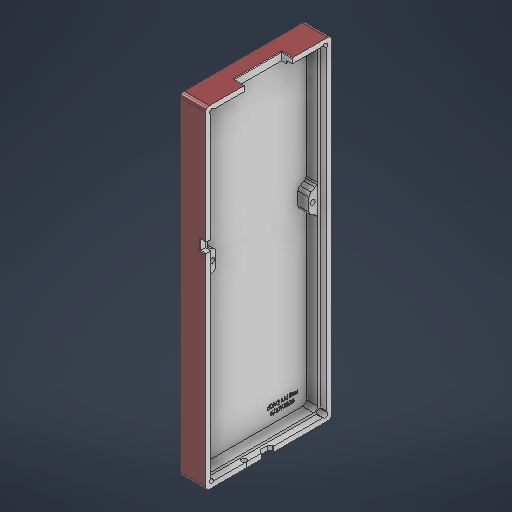
# Autodesk Inventor part: cDAQ_Box_Lid_v0.2
Saved by Autodesk Inventor 2027 (Build 310192000, 192)
## iProperties
Created: 2026-05-08
Part Number: cDAQ_Box_Lid_v0.2
Material: Generic
Document SubType Name: Modeling
Designer: giese
Density: 1 g/cm^3
Appearance: Default
Author: giese
Autodesk Inventor part; units mm, degrees
(part 1 of 2)
ref_plane "YZ Plane" through (0, 0, 0) normal (1, 0, 0) x (0, 1, 0)
ref_plane "XZ Plane" through (0, 0, 0) normal (0, 1, 0) x (-1, 0, 0)
ref_plane "XY Plane" through (0, 0, 0) normal (0, 0, 1) x (1, 0, 0)
sketch "Sketch1" plane through (0, 0, 0) normal (1, 0, 0) x (0, 1, 0)
  line L0 (50.7569, 48.4212) -> (-216.9591, 48.4212)
  line L1 (-216.9591, 48.4212) -> (-216.9591, -53.1788)
  line L2 (-216.9591, -53.1788) -> (50.7569, -53.1788)
  line L3 (50.7569, -53.1788) -> (50.7569, 48.4212)
  point P0 (0, 0)
  dimension "d0" = 101.6
  dimension "d1" = 267.716
  constraints: 8 end point, 2 parallel, 1 horizontal, 1 perpendicular
  measures "d0" distance of L2.end L0.start
  measures "d1" distance of L0.start L0.end
extrude "Extrusion1" add sketch "Sketch1" along normal blind 20.32
sketch "Sketch2" plane through (20.32, 0, 0) normal (1, 0, 0) x (0, 0, -1)
  line L0 (-42.0712, 44.4069) -> (46.8288, 44.4069)
  line L1 (46.8288, 44.4069) -> (46.8288, -210.6091)
  line L2 (46.8288, -210.6091) -> (-42.0712, -210.6091)
  line L3 (-42.0712, -210.6091) -> (-42.0712, 44.4069)
  line L4 (-48.4212, 50.7569) -> (-48.4212, -216.9591) projected
  line L5 (-48.4212, -216.9591) -> (53.1788, -216.9591) projected
  point P0 (0, 0)
  dimension "d4" = 88.9
  dimension "d5" = 255.016
  dimension "d6" = 6.35
  dimension "d7" = 6.35
  constraints: 8 end point, 2 parallel, 1 horizontal, 1 perpendicular
  measures "d4" distance of L0.start L0.end
  measures "d5" distance of L0.end L1.end
  measures "d6" distance between parallel lines of L4 L3
  measures "d7" distance between parallel lines of L5 L2
extrude "Extrusion2" cut sketch "Sketch2" against normal blind 13.97
sketch "Sketch3" plane through (0, 0, 0) normal (-1, 0, 0) x (0, 0, 1)
  circle A0 centre (-30.3188, 7.3229) radius 2
  line L0 (-53.1788, -216.9591) -> (-53.1788, 50.7569) projected
  line L1 (-53.1788, 50.7569) -> (48.4212, 50.7569) projected
  circle A1 centre (-11.82, 7.3229) radius 2
  circle A2 centre (6.6789, 7.3229) radius 2
  point P0 (0, 0)
  dimension "d10" = 22.86
  dimension "d11" = 43.434
  dimension "d12" = 43.434
  dimension "d13" = 18.4988
  dimension "d14" = 4
  dimension "d15" = 4
  dimension "d16" = 43.434
  dimension "d17" = 18.4988
  dimension "d18" = 36.9976
  dimension "d21" = 4
  constraints: 3 centre point
  measures "d10" distance from line of L0 A0.centre
  measures "d11" distance from line of L1 A0.centre
  measures "d12" distance from line of L1 A1.centre
  measures "d13" distance of A0.centre A1.centre
  measures "d14" diameter of A1
  measures "d15" diameter of A2
  measures "d16" distance from line of L1 A2.centre
  measures "d17" distance of A1.centre A2.centre
  measures "d18" distance of A0.centre A2.centre
  measures "d21" diameter of A0
extrude "Extrusion3" [suppressed]
sketch "Sketch6" plane through (0, 50.7569, 48.4212) normal (0, 1, 0) x (1, 0, 0)
  line L0 (20.32, 6.35) -> (20.32, 95.25) projected
  line L1 (11.684, 31.75) -> (20.32, 31.75)
  line L2 (20.32, 31.75) -> (20.32, 69.85)
  line L3 (20.32, 69.85) -> (11.684, 69.85)
  line L4 (11.684, 69.85) -> (11.684, 31.75)
  line L5 (0, 101.6) -> (20.32, 101.6) projected
  point P0 (0, 48.4212)
  point P1 (16.002, 69.85)
  point P2 (16.002, 31.75)
  dimension "d30" = 8.636
  dimension "d31" = 38.1
  dimension "d32" = 31.75
  constraints: 8 end point, 2 midpoint, 2 parallel, 1 horizontal, 1 perpendicular, 1 point on line
  measures "d30" distance between parallel lines of L0 L4
  measures "d31" distance of point (16.002, 69.85) point (16.002, 31.75)
  measures "d32" distance between parallel lines of L5 L3
extrude "Extrusion5" cut sketch "Sketch6" against normal blind 6.35
fillet "Fillet1" radius 3.175 4 edges at (10.16, 50.7569, -53.1788) (10.16, 50.7569, 48.4212) (10.16, -216.9591, 48.4212) (10.16, -216.9591, -53.1788)
sketch "Sketch7" plane through (20.32, 0, 0) normal (1, 0, 0) x (0, 0, -1)
  line L0 (-42.0712, -210.6091) -> (-42.0712, 44.4069) projected
  line L1 (-42.0712, 44.4069) -> (-42.3252, 44.4069)
  line L2 (-42.3252, 46.5659) -> (-44.2302, 46.5659)
  line L3 (-44.2302, 46.5659) -> (-44.2302, 51.0109)
  line L4 (-42.0712, -190.1621) -> (-42.0712, -210.6091)
  line L5 (46.8288, -210.6091) -> (-42.0712, -210.6091) projected
  line L6 (-40.4202, -212.7681) -> (-44.2302, -212.7681)
  line L7 (-44.2302, -212.7681) -> (-44.2302, -190.1621)
  line L8 (46.8288, 44.4069) -> (46.8288, -210.6091) projected
  line L9 (46.8288, -192.7021) -> (46.8288, -210.6091)
  line L10 (46.8288, -210.6091) -> (43.9078, -210.6091)
  line L11 (46.8288, -210.6091) -> (46.8288, -192.7021)
  line L12 (48.9878, -192.7021) -> (48.9878, -212.7681)
  line L13 (48.9878, -212.7681) -> (43.9078, -212.7681)
  line L14 (-42.0712, 44.4069) -> (46.8288, 44.4069) projected
  line L15 (42.0028, 44.4069) -> (46.8288, 44.4069)
  line L16 (48.9878, 48.4709) -> (48.9878, 46.5659)
  line L17 (48.9878, 46.5659) -> (42.0028, 46.5659)
  line L18 (-42.3252, 46.5659) -> (42.0028, 46.5659)
  line L19 (42.0028, 44.4069) -> (-42.3252, 44.4069)
  line L20 (48.9878, 48.4709) -> (48.9878, -192.7021)
  line L21 (44.2888, -195.2421) -> (44.2888, 44.4069)
  line L22 (43.9078, -210.6091) -> (-40.4202, -210.6091)
  line L23 (-40.4202, -212.7681) -> (43.9078, -212.7681)
  line L24 (-44.2302, -190.1621) -> (-44.2302, 51.0109)
  line L25 (-42.0712, 44.4069) -> (-42.0712, -190.1621)
  point P0 (0, 0)
  point P1 (-42.0712, 51.0109)
  point P2 (-44.2302, 48.9789)
  point P3 (46.8288, 48.4709)
  point P4 (48.9878, 46.5659)
  point P5 (-44.2302, 46.5659)
  dimension "d34" = 2.159
  dimension "d35" = 2.159
  dimension "d38" = 2.159
  dimension "d39" = 2.159
  dimension "d42" = 2.159
  dimension "d43" = 2.159
  dimension "d46" = 2.159
  dimension "d47" = 2.159
  constraints: 44 end point, 9 point on line, 4 parallel, 4 perpendicular, 2 collinear, 2 horizontal, 2 vertical
  measures "d34" distance between parallel lines of L2 L1
  measures "d35" distance between parallel lines of L0 L3
  measures "d38" distance between parallel lines of L7 L0
  measures "d39" distance between parallel lines of L5 L6
  measures "d42" distance between parallel lines of L5 L13
  measures "d43" distance between parallel lines of L8 L12
  measures "d46" distance between parallel lines of L14 L17
  measures "d47" distance between parallel lines of L8 L16
extrude "Extrusion6" cut sketch "Sketch7" against normal blind 5 contours L0 L14 L8 L5 | L18 L17 L20 L12 L13 L23 L6 L7 L24 L2
fillet "Fillet2" radius 3.175 6 edges at (10.835, 44.4069, 42.0712) (10.835, 44.4069, -46.8288) (10.835, -210.6091, 42.0712) (17.82, -212.7681, 44.2302) (10.835, -210.6091, -46.8288) (17.82, -212.7681, -48.9878)
sketch "Sketch11" plane through (15.32, 0, 0) normal (1, 0, 0) x (0, 0, -1)
  circle A0 centre (48.0988, 45.6769) radius 1.9939
  line L0 (50.0038, 50.7569) -> (21.4288, 50.7569) projected
  line L1 (53.1788, -213.7841) -> (53.1788, 47.5819) projected
  arc A1 (46.9238, 45.7719) -> (43.7488, 48.9469) centre (43.7488, 45.7719) ccw projected
  circle A2 centre (-43.3412, 45.6769) radius 1.9939
  line L2 (-48.4212, 47.5819) -> (-48.4212, -213.7841) projected
  line L3 (-16.6712, 50.7569) -> (-45.2462, 50.7569) projected
  circle A3 centre (48.0988, -211.8791) radius 1.9939
  line L4 (-45.2462, -216.9591) -> (50.0038, -216.9591) projected
  circle A4 centre (-43.3412, -211.8791) radius 1.9939
  circle A5 centre (43.0188, -63.5431) radius 1.9939
  circle A6 centre (-38.2612, -63.5431) radius 1.9939
  point P0 (0, 0)
  point P1 (45.9939, 48.017)
  point P2 (48.5528, -43.2993)
  point P3 (45.3778, -46.4743)
  point P4 (-30.4007, -42.8803)
  point P5 (-33.5757, -46.0553)
  dimension "d58" = 3.9878
  dimension "d59" = 5.08
  dimension "d60" = 5.08
  dimension "d61" = 3.9878
  dimension "d62" = 3.9878
  dimension "d63" = 5.08
  dimension "d64" = 5.08
  dimension "d65" = 3.9878
  dimension "d66" = 5.08
  dimension "d67" = 5.08
  dimension "d76" = 5.08
  dimension "d77" = 5.08
  dimension "d114" = 3.9878
  dimension "d115" = 114.3
  dimension "d116" = 10.16
  dimension "d117" = 3.9878
  dimension "d118" = 114.3
  dimension "d119" = 10.16
  constraints: 6 centre point, 1 point on circle
  measures "d58" diameter of A0
  measures "d59" distance from line of L2 A2.centre
  measures "d60" distance from line of L3 A2.centre
  measures "d61" diameter of A2
  measures "d62" diameter of A3
  measures "d63" distance from line of L1 A3.centre
  measures "d64" distance from line of L4 A3.centre
  measures "d65" diameter of A4
  measures "d66" distance from line of L2 A4.centre
  measures "d67" distance from line of L4 A4.centre
  measures "d76" distance from line of L1 A0.centre
  measures "d77" distance from line of L0 A0.centre
  measures "d114" diameter of A5
  measures "d115" distance from line of A5.centre L0
  measures "d116" distance from line of L1 A5.centre
  measures "d117" diameter of A6
  measures "d118" distance from line of A6.centre L3
  measures "d119" distance from line of L2 A6.centre
extrude "Extrusion8" cut sketch "Sketch11" along normal blind 5.08 and the other way blind 17.78
sketch "Sketch13" plane through (6.35, 0, 0) normal (1, 0, 0) x (0, 0, -1)
  line L0 (14.9448, -196.2811) -> (40.0007, -196.2811) construction
  line L1 (40.0007, -196.2811) -> (40.0007, -205.1454) construction
  line L2 (40.0007, -205.1454) -> (14.9448, -205.1454) construction
  line L3 (14.9448, -205.1454) -> (14.9448, -196.2811) construction
  spline S0 degree 2 poles (16.1329, -199.5168) (15.8958, -199.5168) (15.5031, -199.3711) (15.3623, -199.2229) knots 0 0 0 1 2 2 2
  spline S1 degree 2 poles (15.3623, -199.2229) (15.2215, -199.0772) (15.0659, -198.6276) (15.0659, -198.3263) knots 0 0 0 1 2 2 2
  spline S2 degree 2 poles (15.0659, -198.3263) (15.0659, -198.0249) (15.2264, -197.5853) (15.3623, -197.4371) knots 0 0 0 1 2 2 2
  spline S3 degree 2 poles (15.3623, -197.4371) (15.4981, -197.2864) (15.9007, -197.1258) (16.1329, -197.1258) knots 0 0 0 1 2 2 2
  spline S4 degree 2 poles (16.1329, -197.1258) (16.3206, -197.1258) (16.6714, -197.232) (16.8072, -197.3012) knots 0 0 0 1 2 2 2
  line L4 (16.8072, -197.3012) -> (16.8072, -197.7335)
  line L5 (16.8072, -197.7335) -> (16.785, -197.7335)
  spline S5 degree 2 poles (16.785, -197.7335) (16.743, -197.6989) (16.6146, -197.61) (16.5232, -197.563) knots 0 0 0 1 2 2 2
  spline S6 degree 2 poles (16.5232, -197.563) (16.4417, -197.5235) (16.2243, -197.4618) (16.1255, -197.4618) knots 0 0 0 1 2 2 2
  spline S7 degree 2 poles (16.1255, -197.4618) (15.8266, -197.4618) (15.4635, -197.9138) (15.4635, -198.3263) knots 0 0 0 1 2 2 2
  spline S8 degree 2 poles (15.4635, -198.3263) (15.4635, -198.7289) (15.8143, -199.1809) (16.1255, -199.1809) knots 0 0 0 1 2 2 2
  spline S9 degree 2 poles (16.1255, -199.1809) (16.3132, -199.1809) (16.6541, -199.0253) (16.785, -198.9043) knots 0 0 0 1 2 2 2
  line L6 (16.785, -198.9043) -> (16.8072, -198.9043)
  line L7 (16.8072, -198.9043) -> (16.8072, -199.3365)
  spline S10 degree 2 poles (16.8072, -199.3365) (16.7504, -199.3637) (16.5775, -199.4402) (16.5084, -199.4575) knots 0 0 0 1 2 2 2
  spline S11 degree 2 poles (16.5084, -199.4575) (16.4096, -199.4872) (16.2539, -199.5168) (16.1329, -199.5168) knots 0 0 0 1 2 2 2
  spline S12 degree 2 poles (19.5909, -197.9434) (19.5909, -198.3608) (19.2525, -199.0327) (18.9685, -199.2204) knots 0 0 0 1 2 2 2
  spline S13 degree 2 poles (18.9685, -199.2204) (18.7363, -199.3661) (18.2596, -199.4649) (17.8891, -199.4649) knots 0 0 0 1 2 2 2
  line L8 (17.8891, -199.4649) -> (17.1876, -199.4649)
  line L9 (17.1876, -199.4649) -> (17.1876, -196.4169)
  line L10 (17.1876, -196.4169) -> (17.8817, -196.4169)
  spline S14 degree 2 poles (17.8817, -196.4169) (18.3115, -196.4169) (18.8005, -196.5454) (18.9734, -196.659) knots 0 0 0 1 2 2 2
  spline S15 degree 2 poles (18.9734, -196.659) (19.2674, -196.8541) (19.5909, -197.4988) (19.5909, -197.9434) knots 0 0 0 1 2 2 2
  spline S16 degree 2 poles (19.1686, -197.9385) (19.1686, -197.5877) (18.9364, -197.0913) (18.7067, -196.9505) knots 0 0 0 1 2 2 2
  spline S17 degree 2 poles (18.7067, -196.9505) (18.5437, -196.8541) (18.1756, -196.7677) (17.9014, -196.7677) knots 0 0 0 1 2 2 2
  line L11 (17.9014, -196.7677) -> (17.5927, -196.7677)
  line L12 (17.5927, -196.7677) -> (17.5927, -199.1142)
  line L13 (17.5927, -199.1142) -> (17.9014, -199.1142)
  spline S18 degree 2 poles (17.9014, -199.1142) (18.1707, -199.1142) (18.5782, -199.0278) (18.7437, -198.9117) knots 0 0 0 1 2 2 2
  spline S19 degree 2 poles (18.7437, -198.9117) (18.9561, -198.7684) (19.1686, -198.2942) (19.1686, -197.9385) knots 0 0 0 1 2 2 2
  line L14 (19.7021, -199.4649) -> (20.7296, -196.4169)
  line L15 (20.7296, -196.4169) -> (21.2286, -196.4169)
  line L16 (21.2286, -196.4169) -> (22.2561, -199.4649)
  line L17 (22.2561, -199.4649) -> (21.8288, -199.4649)
  line L18 (21.8288, -199.4649) -> (21.5521, -198.6128)
  line L19 (21.5521, -198.6128) -> (20.3888, -198.6128)
  line L20 (20.3888, -198.6128) -> (20.1121, -199.4649)
  line L21 (20.1121, -199.4649) -> (19.7021, -199.4649)
  line L22 (21.441, -198.267) -> (20.9692, -196.8319)
  line L23 (20.9692, -196.8319) -> (20.4999, -198.267)
  line L24 (20.4999, -198.267) -> (21.441, -198.267)
  spline S20 degree 2 poles (25.0768, -200.2109) (24.9657, -200.2381) (24.7236, -200.2677) (24.6026, -200.2677) knots 0 0 0 1 2 2 2
  spline S21 degree 2 poles (24.6026, -200.2677) (24.2593, -200.2677) (23.832, -199.8848) (23.8122, -199.5292) knots 0 0 0 1 2 2 2
  spline S22 degree 2 poles (23.8122, -199.5292) (23.785, -199.5292) (23.7381, -199.5292) (23.7183, -199.5292) knots 0 0 0 1 2 2 2
  spline S23 degree 2 poles (23.7183, -199.5292) (23.4096, -199.5292) (22.9131, -199.3192) (22.7353, -199.1142) knots 0 0 0 1 2 2 2
  spline S24 degree 2 poles (22.7353, -199.1142) (22.5599, -198.9117) (22.3722, -198.3189) (22.3722, -197.9434) knots 0 0 0 1 2 2 2
  spline S25 degree 2 poles (22.3722, -197.9434) (22.3722, -197.5581) (22.5624, -196.9752) (22.7377, -196.7677) knots 0 0 0 1 2 2 2
  spline S26 degree 2 poles (22.7377, -196.7677) (22.9156, -196.5627) (23.4121, -196.3527) (23.7183, -196.3527) knots 0 0 0 1 2 2 2
  spline S27 degree 2 poles (23.7183, -196.3527) (24.0296, -196.3527) (24.5285, -196.5701) (24.7014, -196.7677) knots 0 0 0 1 2 2 2
  spline S28 degree 2 poles (24.7014, -196.7677) (24.8743, -196.9678) (25.067, -197.563) (25.067, -197.9434) knots 0 0 0 1 2 2 2
  spline S29 degree 2 poles (25.067, -197.9434) (25.067, -198.5362) (24.6051, -199.3069) (24.2025, -199.4427) knots 0 0 0 1 2 2 2
  spline S30 degree 2 poles (24.2025, -199.4427) (24.2123, -199.5563) (24.2716, -199.7391) (24.3185, -199.791) knots 0 0 0 1 2 2 2
  spline S31 degree 2 poles (24.3185, -199.791) (24.3754, -199.8552) (24.531, -199.9145) (24.6693, -199.9145) knots 0 0 0 1 2 2 2
  spline S32 degree 2 poles (24.6693, -199.9145) (24.7508, -199.9145) (24.9731, -199.8626) (25.0225, -199.8429) knots 0 0 0 1 2 2 2
  line L25 (25.0225, -199.8429) -> (25.0768, -199.8429)
  line L26 (25.0768, -199.8429) -> (25.0768, -200.2109)
  spline S33 degree 2 poles (24.6446, -197.9434) (24.6446, -197.6396) (24.5137, -197.1728) (24.3951, -197.0196) knots 0 0 0 1 2 2 2
  spline S34 degree 2 poles (24.3951, -197.0196) (24.2741, -196.8615) (23.9332, -196.7035) (23.7208, -196.7035) knots 0 0 0 1 2 2 2
  spline S35 degree 2 poles (23.7208, -196.7035) (23.501, -196.7035) (23.17, -196.8566) (23.044, -197.0196) knots 0 0 0 1 2 2 2
  spline S36 degree 2 poles (23.044, -197.0196) (22.923, -197.1752) (22.7945, -197.647) (22.7945, -197.9434) knots 0 0 0 1 2 2 2
  spline S37 degree 2 poles (22.7945, -197.9434) (22.7945, -198.5436) (23.2984, -199.1834) (23.7208, -199.1834) knots 0 0 0 1 2 2 2
  spline S38 degree 2 poles (23.7208, -199.1834) (24.1432, -199.1834) (24.6446, -198.5436) (24.6446, -197.9434) knots 0 0 0 1 2 2 2
  line L27 (28.5867, -199.4649) -> (26.8207, -199.4649)
  line L28 (26.8207, -199.4649) -> (26.8207, -196.4169)
  line L29 (26.8207, -196.4169) -> (27.2258, -196.4169)
  line L30 (27.2258, -196.4169) -> (27.2258, -199.1043)
  line L31 (27.2258, -199.1043) -> (28.5867, -199.1043)
  line L32 (28.5867, -199.1043) -> (28.5867, -199.4649)
  line L33 (29.2685, -199.4649) -> (28.8831, -199.4649)
  line L34 (28.8831, -199.4649) -> (28.8831, -197.1777)
  line L35 (28.8831, -197.1777) -> (29.2685, -197.1777)
  line L36 (29.2685, -197.1777) -> (29.2685, -199.4649)
  line L37 (29.2956, -196.7973) -> (28.8584, -196.7973)
  line L38 (28.8584, -196.7973) -> (28.8584, -196.3972)
  line L39 (28.8584, -196.3972) -> (29.2956, -196.3972)
  line L40 (29.2956, -196.3972) -> (29.2956, -196.7973)
  line L41 (31.5927, -199.4649) -> (31.2074, -199.4649)
  line L42 (31.2074, -199.4649) -> (31.2074, -199.2328)
  spline S39 degree 2 poles (31.2074, -199.2328) (31.1185, -199.3069) (30.9876, -199.4057) (30.8987, -199.4477) knots 0 0 0 1 2 2 2
  spline S40 degree 2 poles (30.8987, -199.4477) (30.8172, -199.4872) (30.6418, -199.5292) (30.5257, -199.5292) knots 0 0 0 1 2 2 2
  spline S41 degree 2 poles (30.5257, -199.5292) (30.338, -199.5292) (30.0218, -199.3736) (29.9107, -199.2229) knots 0 0 0 1 2 2 2
  spline S42 degree 2 poles (29.9107, -199.2229) (29.7995, -199.0722) (29.676, -198.6276) (29.676, -198.3386) knots 0 0 0 1 2 2 2
  spline S43 degree 2 poles (29.676, -198.3386) (29.676, -198.0373) (29.8316, -197.5976) (29.9675, -197.4321) knots 0 0 0 1 2 2 2
  spline S44 degree 2 poles (29.9675, -197.4321) (30.0934, -197.2839) (30.4467, -197.1135) (30.6418, -197.1135) knots 0 0 0 1 2 2 2
  spline S45 degree 2 poles (30.6418, -197.1135) (30.8122, -197.1135) (31.0666, -197.1901) (31.2074, -197.2691) knots 0 0 0 1 2 2 2
  line L43 (31.2074, -197.2691) -> (31.2074, -196.2811)
  line L44 (31.2074, -196.2811) -> (31.5927, -196.2811)
  line L45 (31.5927, -196.2811) -> (31.5927, -199.4649)
  line L46 (31.2074, -198.9092) -> (31.2074, -197.5877)
  spline S46 degree 2 poles (31.2074, -197.5877) (31.0642, -197.5186) (30.8369, -197.4667) (30.706, -197.4667) knots 0 0 0 1 2 2 2
  spline S47 degree 2 poles (30.706, -197.4667) (30.4096, -197.4667) (30.0737, -197.9113) (30.0737, -198.3312) knots 0 0 0 1 2 2 2
  spline S48 degree 2 poles (30.0737, -198.3312) (30.0737, -198.7363) (30.3306, -199.1636) (30.6146, -199.1636) knots 0 0 0 1 2 2 2
  spline S49 degree 2 poles (30.6146, -199.1636) (30.7653, -199.1636) (31.0716, -199.0253) (31.2074, -198.9092) knots 0 0 0 1 2 2 2
  spline S50 degree 2 poles (35.5571, -198.5288) (35.5571, -198.756) (35.3842, -199.1043) (35.241, -199.2179) knots 0 0 0 1 2 2 2
  spline S51 degree 2 poles (35.241, -199.2179) (35.0681, -199.3513) (34.6753, -199.4649) (34.3641, -199.4649) knots 0 0 0 1 2 2 2
  line L47 (34.3641, -199.4649) -> (33.4897, -199.4649)
  line L48 (33.4897, -199.4649) -> (33.4897, -196.4169)
  line L49 (33.4897, -196.4169) -> (34.2974, -196.4169)
  spline S52 degree 2 poles (34.2974, -196.4169) (34.6235, -196.4169) (34.9495, -196.4589) (35.0977, -196.5404) knots 0 0 0 1 2 2 2
  spline S53 degree 2 poles (35.0977, -196.5404) (35.2632, -196.6269) (35.4139, -196.9109) (35.4139, -197.1036) knots 0 0 0 1 2 2 2
  spline S54 degree 2 poles (35.4139, -197.1036) (35.4139, -197.3185) (35.1866, -197.6594) (34.9865, -197.7557) knots 0 0 0 1 2 2 2
  line L50 (34.9865, -197.7557) -> (34.9865, -197.7705)
  spline S55 degree 2 poles (34.9865, -197.7705) (35.2583, -197.8446) (35.5571, -198.2373) (35.5571, -198.5288) knots 0 0 0 1 2 2 2
  spline S56 degree 2 poles (35.1347, -198.5461) (35.1347, -198.3732) (35.0359, -198.1509) (34.8877, -198.0719) knots 0 0 0 1 2 2 2
  spline S57 degree 2 poles (34.8877, -198.0719) (34.7914, -198.0225) (34.5642, -197.9928) (34.3542, -197.9928) knots 0 0 0 1 2 2 2
  line L51 (34.3542, -197.9928) -> (33.8948, -197.9928)
  line L52 (33.8948, -197.9928) -> (33.8948, -199.1191)
  line L53 (33.8948, -199.1191) -> (34.2233, -199.1191)
  spline S58 degree 2 poles (34.2233, -199.1191) (34.4901, -199.1191) (34.7964, -199.0697) (34.9149, -198.9907) knots 0 0 0 1 2 2 2
  spline S59 degree 2 poles (34.9149, -198.9907) (35.0285, -198.9092) (35.1347, -198.7066) (35.1347, -198.5461) knots 0 0 0 1 2 2 2
  spline S60 degree 2 poles (34.9915, -197.1604) (34.9915, -197.0517) (34.9174, -196.8887) (34.8359, -196.8418) knots 0 0 0 1 2 2 2
  spline S61 degree 2 poles (34.8359, -196.8418) (34.7371, -196.7874) (34.4975, -196.7627) (34.2826, -196.7627) knots 0 0 0 1 2 2 2
  line L54 (34.2826, -196.7627) -> (33.8948, -196.7627)
  line L55 (33.8948, -196.7627) -> (33.8948, -197.6544)
  line L56 (33.8948, -197.6544) -> (34.3542, -197.6544)
  spline S62 degree 2 poles (34.3542, -197.6544) (34.5444, -197.6544) (34.7247, -197.6149) (34.8211, -197.5532) knots 0 0 0 1 2 2 2
  spline S63 degree 2 poles (34.8211, -197.5532) (34.9149, -197.4939) (34.9915, -197.3037) (34.9915, -197.1604) knots 0 0 0 1 2 2 2
  spline S64 degree 2 poles (37.8098, -198.3213) (37.8098, -198.8993) (37.254, -199.5292) (36.7897, -199.5292) knots 0 0 0 1 2 2 2
  spline S65 degree 2 poles (36.7897, -199.5292) (36.3129, -199.5292) (35.7671, -198.8796) (35.7671, -198.3213) knots 0 0 0 1 2 2 2
  spline S66 degree 2 poles (35.7671, -198.3213) (35.7671, -197.7483) (36.3302, -197.1135) (36.7897, -197.1135) knots 0 0 0 1 2 2 2
  spline S67 degree 2 poles (36.7897, -197.1135) (37.254, -197.1135) (37.8098, -197.7458) (37.8098, -198.3213) knots 0 0 0 1 2 2 2
  spline S68 degree 2 poles (37.4121, -198.3213) (37.4121, -197.8767) (37.0885, -197.4445) (36.7897, -197.4445) knots 0 0 0 1 2 2 2
  spline S69 degree 2 poles (36.7897, -197.4445) (36.4908, -197.4445) (36.1647, -197.8767) (36.1647, -198.3213) knots 0 0 0 1 2 2 2
  spline S70 degree 2 poles (36.1647, -198.3213) (36.1647, -198.7536) (36.4908, -199.1982) (36.7897, -199.1982) knots 0 0 0 1 2 2 2
  spline S71 degree 2 poles (36.7897, -199.1982) (37.0861, -199.1982) (37.4121, -198.761) (37.4121, -198.3213) knots 0 0 0 1 2 2 2
  line L57 (39.9809, -199.4649) -> (39.5091, -199.4649)
  line L58 (39.5091, -199.4649) -> (38.9534, -198.6054)
  line L59 (38.9534, -198.6054) -> (38.3828, -199.4649)
  line L60 (38.3828, -199.4649) -> (37.9456, -199.4649)
  line L61 (37.9456, -199.4649) -> (38.7385, -198.3312)
  line L62 (38.7385, -198.3312) -> (37.953, -197.1777)
  line L63 (37.953, -197.1777) -> (38.4248, -197.1777)
  line L64 (38.4248, -197.1777) -> (38.9781, -198.0299)
  line L65 (38.9781, -198.0299) -> (39.5437, -197.1777)
  line L66 (39.5437, -197.1777) -> (39.9809, -197.1777)
  line L67 (39.9809, -197.1777) -> (39.193, -198.3065)
  line L68 (39.193, -198.3065) -> (39.9809, -199.4649)
  spline S72 degree 2 poles (20.0133, -203.4954) (20.0133, -203.73) (19.8577, -204.1277) (19.7268, -204.2611) knots 0 0 0 1 2 2 2
  spline S73 degree 2 poles (19.7268, -204.2611) (19.5909, -204.4019) (19.2501, -204.5476) (19.0451, -204.5476) knots 0 0 0 1 2 2 2
  spline S74 degree 2 poles (19.0451, -204.5476) (18.8401, -204.5476) (18.5017, -204.4093) (18.3732, -204.271) knots 0 0 0 1 2 2 2
  spline S75 degree 2 poles (18.3732, -204.271) (18.2151, -204.1055) (18.0373, -203.5497) (18.0373, -203.1446) knots 0 0 0 1 2 2 2
  spline S76 degree 2 poles (18.0373, -203.1446) (18.0373, -202.747) (18.2003, -202.1072) (18.3707, -201.8701) knots 0 0 0 1 2 2 2
  spline S77 degree 2 poles (18.3707, -201.8701) (18.5362, -201.6379) (19.0599, -201.3786) (19.4032, -201.3786) knots 0 0 0 1 2 2 2
  spline S78 degree 2 poles (19.4032, -201.3786) (19.5045, -201.3786) (19.6823, -201.3983) (19.749, -201.4206) knots 0 0 0 1 2 2 2
  line L69 (19.749, -201.4206) -> (19.749, -201.8133)
  line L70 (19.749, -201.8133) -> (19.7317, -201.8133)
  spline S79 degree 2 poles (19.7317, -201.8133) (19.6749, -201.7837) (19.4674, -201.7318) (19.3489, -201.7318) knots 0 0 0 1 2 2 2
  spline S80 degree 2 poles (19.3489, -201.7318) (18.9685, -201.7318) (18.5017, -202.2456) (18.4572, -202.7494) knots 0 0 0 1 2 2 2
  spline S81 degree 2 poles (18.4572, -202.7494) (18.6029, -202.6482) (18.9092, -202.537) (19.092, -202.537) knots 0 0 0 1 2 2 2
  spline S82 degree 2 poles (19.092, -202.537) (19.2698, -202.537) (19.5366, -202.6087) (19.6823, -202.7173) knots 0 0 0 1 2 2 2
  spline S83 degree 2 poles (19.6823, -202.7173) (19.8503, -202.8433) (20.0133, -203.2336) (20.0133, -203.4954) knots 0 0 0 1 2 2 2
  spline S84 degree 2 poles (19.5983, -203.5127) (19.5983, -203.325) (19.4995, -203.0705) (19.3909, -202.9816) knots 0 0 0 1 2 2 2
  spline S85 degree 2 poles (19.3909, -202.9816) (19.3094, -202.9174) (19.1068, -202.8754) (19.0006, -202.8754) knots 0 0 0 1 2 2 2
  spline S86 degree 2 poles (19.0006, -202.8754) (18.8573, -202.8754) (18.5881, -202.9619) (18.4572, -203.0434) knots 0 0 0 1 2 2 2
  spline S87 degree 2 poles (18.4572, -203.0434) (18.4547, -203.0878) (18.4498, -203.1718) (18.4498, -203.236) knots 0 0 0 1 2 2 2
  spline S88 degree 2 poles (18.4498, -203.236) (18.4498, -203.5522) (18.5733, -203.94) (18.6672, -204.0413) knots 0 0 0 1 2 2 2
  spline S89 degree 2 poles (18.6672, -204.0413) (18.7536, -204.1376) (18.9413, -204.2142) (19.0475, -204.2142) knots 0 0 0 1 2 2 2
  spline S90 degree 2 poles (19.0475, -204.2142) (19.2945, -204.2142) (19.5983, -203.8634) (19.5983, -203.5127) knots 0 0 0 1 2 2 2
  line L71 (21.6411, -201.2995) -> (20.448, -205.1454)
  line L72 (20.448, -205.1454) -> (20.1022, -205.1454)
  line L73 (20.1022, -205.1454) -> (21.2903, -201.2995)
  line L74 (21.2903, -201.2995) -> (21.6411, -201.2995)
  line L75 (23.7035, -204.4834) -> (22.2166, -204.4834)
  line L76 (22.2166, -204.4834) -> (22.2166, -204.1722)
  line L77 (22.2166, -204.1722) -> (22.7698, -204.1722)
  line L78 (22.7698, -204.1722) -> (22.7698, -202.1295)
  line L79 (22.7698, -202.1295) -> (22.2166, -202.1295)
  line L80 (22.2166, -202.1295) -> (22.2166, -201.8504)
  spline S91 degree 2 poles (22.2166, -201.8504) (22.5303, -201.8504) (22.8267, -201.6725) (22.8464, -201.4255) knots 0 0 0 1 2 2 2
  line L81 (22.8464, -201.4255) -> (23.1626, -201.4255)
  line L82 (23.1626, -201.4255) -> (23.1626, -204.1722)
  line L83 (23.1626, -204.1722) -> (23.7035, -204.1722)
  line L84 (23.7035, -204.1722) -> (23.7035, -204.4834)
  line L85 (26.1785, -201.8923) -> (24.8595, -204.4834)
  line L86 (24.8595, -204.4834) -> (24.4248, -204.4834)
  line L87 (24.4248, -204.4834) -> (25.8178, -201.7935)
  line L88 (25.8178, -201.7935) -> (24.2444, -201.7935)
  line L89 (24.2444, -201.7935) -> (24.2444, -201.4354)
  line L90 (24.2444, -201.4354) -> (26.1785, -201.4354)
  line L91 (26.1785, -201.4354) -> (26.1785, -201.8923)
  line L92 (27.8186, -201.2995) -> (26.6255, -205.1454)
  line L93 (26.6255, -205.1454) -> (26.2797, -205.1454)
  line L94 (26.2797, -205.1454) -> (27.4678, -201.2995)
  line L95 (27.4678, -201.2995) -> (27.8186, -201.2995)
  line L96 (30.0342, -204.4834) -> (28.1545, -204.4834)
  line L97 (28.1545, -204.4834) -> (28.1545, -204.0511)
  spline S92 degree 2 poles (28.1545, -204.0511) (28.357, -203.861) (28.7176, -203.5077) (28.8905, -203.3175) knots 0 0 0 1 2 2 2
  spline S93 degree 2 poles (28.8905, -203.3175) (29.2388, -202.9347) (29.4932, -202.4753) (29.4932, -202.2307) knots 0 0 0 1 2 2 2
  spline S94 degree 2 poles (29.4932, -202.2307) (29.4932, -202.1023) (29.4142, -201.9096) (29.3426, -201.8479) knots 0 0 0 1 2 2 2
  spline S95 degree 2 poles (29.3426, -201.8479) (29.2709, -201.7861) (29.0832, -201.7244) (28.9696, -201.7244) knots 0 0 0 1 2 2 2
  spline S96 degree 2 poles (28.9696, -201.7244) (28.8609, -201.7244) (28.6386, -201.7787) (28.5373, -201.8207) knots 0 0 0 1 2 2 2
  spline S97 degree 2 poles (28.5373, -201.8207) (28.4509, -201.8553) (28.2903, -201.9541) (28.2409, -201.9887) knots 0 0 0 1 2 2 2
  line L98 (28.2409, -201.9887) -> (28.2187, -201.9887)
  line L99 (28.2187, -201.9887) -> (28.2187, -201.554)
  spline S98 degree 2 poles (28.2187, -201.554) (28.3447, -201.4922) (28.7967, -201.3712) (28.9992, -201.3712) knots 0 0 0 1 2 2 2
  spline S99 degree 2 poles (28.9992, -201.3712) (29.4265, -201.3712) (29.9082, -201.8232) (29.9082, -202.2085) knots 0 0 0 1 2 2 2
  spline S100 degree 2 poles (29.9082, -202.2085) (29.9082, -202.3888) (29.8242, -202.6902) (29.7501, -202.8186) knots 0 0 0 1 2 2 2
  spline S101 degree 2 poles (29.7501, -202.8186) (29.676, -202.952) (29.4611, -203.2138) (29.3426, -203.3398) knots 0 0 0 1 2 2 2
  spline S102 degree 2 poles (29.3426, -203.3398) (29.1499, -203.5497) (28.6781, -203.9993) (28.5373, -204.1302) knots 0 0 0 1 2 2 2
  line L100 (28.5373, -204.1302) -> (30.0342, -204.1302)
  line L101 (30.0342, -204.1302) -> (30.0342, -204.4834)
  spline S103 degree 2 poles (32.3387, -202.9594) (32.3387, -203.7794) (31.862, -204.5476) (31.3655, -204.5476) knots 0 0 0 1 2 2 2
  spline S104 degree 2 poles (31.3655, -204.5476) (30.8616, -204.5476) (30.3898, -203.7646) (30.3898, -202.9619) knots 0 0 0 1 2 2 2
  spline S105 degree 2 poles (30.3898, -202.9619) (30.3898, -202.1369) (30.8666, -201.3736) (31.3655, -201.3736) knots 0 0 0 1 2 2 2
  spline S106 degree 2 poles (31.3655, -201.3736) (31.8669, -201.3736) (32.3387, -202.1641) (32.3387, -202.9594) knots 0 0 0 1 2 2 2
  spline S107 degree 2 poles (31.815, -203.8881) (31.8743, -203.7375) (31.9237, -203.2731) (31.9237, -202.9594) knots 0 0 0 1 2 2 2
  spline S108 degree 2 poles (31.9237, -202.9594) (31.9237, -202.6457) (31.8743, -202.1838) (31.8126, -202.0282) knots 0 0 0 1 2 2 2
  spline S109 degree 2 poles (31.8126, -202.0282) (31.7508, -201.8726) (31.5359, -201.712) (31.3655, -201.712) knots 0 0 0 1 2 2 2
  spline S110 degree 2 poles (31.3655, -201.712) (31.1951, -201.712) (30.9752, -201.8726) (30.911, -202.0331) knots 0 0 0 1 2 2 2
  spline S111 degree 2 poles (30.911, -202.0331) (30.8493, -202.1888) (30.8048, -202.663) (30.8048, -202.9619) knots 0 0 0 1 2 2 2
  spline S112 degree 2 poles (30.8048, -202.9619) (30.8048, -203.283) (30.8443, -203.7128) (30.9086, -203.8807) knots 0 0 0 1 2 2 2
  spline S113 degree 2 poles (30.9086, -203.8807) (30.9678, -204.0388) (31.1877, -204.2092) (31.3655, -204.2092) knots 0 0 0 1 2 2 2
  spline S114 degree 2 poles (31.3655, -204.2092) (31.5335, -204.2092) (31.7533, -204.0487) (31.815, -203.8881) knots 0 0 0 1 2 2 2
  line L102 (34.6086, -204.4834) -> (32.729, -204.4834)
  line L103 (32.729, -204.4834) -> (32.729, -204.0511)
  spline S115 degree 2 poles (32.729, -204.0511) (32.9315, -203.861) (33.2921, -203.5077) (33.465, -203.3175) knots 0 0 0 1 2 2 2
  spline S116 degree 2 poles (33.465, -203.3175) (33.8133, -202.9347) (34.0677, -202.4753) (34.0677, -202.2307) knots 0 0 0 1 2 2 2
  spline S117 degree 2 poles (34.0677, -202.2307) (34.0677, -202.1023) (33.9887, -201.9096) (33.917, -201.8479) knots 0 0 0 1 2 2 2
  spline S118 degree 2 poles (33.917, -201.8479) (33.8454, -201.7861) (33.6577, -201.7244) (33.5441, -201.7244) knots 0 0 0 1 2 2 2
  spline S119 degree 2 poles (33.5441, -201.7244) (33.4354, -201.7244) (33.2131, -201.7787) (33.1118, -201.8207) knots 0 0 0 1 2 2 2
  spline S120 degree 2 poles (33.1118, -201.8207) (33.0254, -201.8553) (32.8648, -201.9541) (32.8154, -201.9887) knots 0 0 0 1 2 2 2
  line L104 (32.8154, -201.9887) -> (32.7932, -201.9887)
  line L105 (32.7932, -201.9887) -> (32.7932, -201.554)
  spline S121 degree 2 poles (32.7932, -201.554) (32.9191, -201.4922) (33.3712, -201.3712) (33.5737, -201.3712) knots 0 0 0 1 2 2 2
  spline S122 degree 2 poles (33.5737, -201.3712) (34.001, -201.3712) (34.4827, -201.8232) (34.4827, -202.2085) knots 0 0 0 1 2 2 2
  spline S123 degree 2 poles (34.4827, -202.2085) (34.4827, -202.3888) (34.3987, -202.6902) (34.3246, -202.8186) knots 0 0 0 1 2 2 2
  spline S124 degree 2 poles (34.3246, -202.8186) (34.2505, -202.952) (34.0356, -203.2138) (33.917, -203.3398) knots 0 0 0 1 2 2 2
  spline S125 degree 2 poles (33.917, -203.3398) (33.7244, -203.5497) (33.2526, -203.9993) (33.1118, -204.1302) knots 0 0 0 1 2 2 2
  line L106 (33.1118, -204.1302) -> (34.6086, -204.1302)
  line L107 (34.6086, -204.1302) -> (34.6086, -204.4834)
  spline S126 degree 2 poles (36.9428, -203.4954) (36.9428, -203.73) (36.7872, -204.1277) (36.6563, -204.2611) knots 0 0 0 1 2 2 2
  spline S127 degree 2 poles (36.6563, -204.2611) (36.5204, -204.4019) (36.1796, -204.5476) (35.9746, -204.5476) knots 0 0 0 1 2 2 2
  spline S128 degree 2 poles (35.9746, -204.5476) (35.7695, -204.5476) (35.4312, -204.4093) (35.3027, -204.271) knots 0 0 0 1 2 2 2
  spline S129 degree 2 poles (35.3027, -204.271) (35.1446, -204.1055) (34.9668, -203.5497) (34.9668, -203.1446) knots 0 0 0 1 2 2 2
  spline S130 degree 2 poles (34.9668, -203.1446) (34.9668, -202.747) (35.1298, -202.1072) (35.3002, -201.8701) knots 0 0 0 1 2 2 2
  spline S131 degree 2 poles (35.3002, -201.8701) (35.4657, -201.6379) (35.9894, -201.3786) (36.3327, -201.3786) knots 0 0 0 1 2 2 2
  spline S132 degree 2 poles (36.3327, -201.3786) (36.434, -201.3786) (36.6118, -201.3983) (36.6785, -201.4206) knots 0 0 0 1 2 2 2
  line L108 (36.6785, -201.4206) -> (36.6785, -201.8133)
  line L109 (36.6785, -201.8133) -> (36.6612, -201.8133)
  spline S133 degree 2 poles (36.6612, -201.8133) (36.6044, -201.7837) (36.3969, -201.7318) (36.2784, -201.7318) knots 0 0 0 1 2 2 2
  spline S134 degree 2 poles (36.2784, -201.7318) (35.898, -201.7318) (35.4312, -202.2456) (35.3867, -202.7494) knots 0 0 0 1 2 2 2
  spline S135 degree 2 poles (35.3867, -202.7494) (35.5324, -202.6482) (35.8387, -202.537) (36.0215, -202.537) knots 0 0 0 1 2 2 2
  spline S136 degree 2 poles (36.0215, -202.537) (36.1993, -202.537) (36.4661, -202.6087) (36.6118, -202.7173) knots 0 0 0 1 2 2 2
  spline S137 degree 2 poles (36.6118, -202.7173) (36.7798, -202.8433) (36.9428, -203.2336) (36.9428, -203.4954) knots 0 0 0 1 2 2 2
  spline S138 degree 2 poles (36.5278, -203.5127) (36.5278, -203.325) (36.429, -203.0705) (36.3204, -202.9816) knots 0 0 0 1 2 2 2
  spline S139 degree 2 poles (36.3204, -202.9816) (36.2388, -202.9174) (36.0363, -202.8754) (35.9301, -202.8754) knots 0 0 0 1 2 2 2
  spline S140 degree 2 poles (35.9301, -202.8754) (35.7868, -202.8754) (35.5176, -202.9619) (35.3867, -203.0434) knots 0 0 0 1 2 2 2
  spline S141 degree 2 poles (35.3867, -203.0434) (35.3842, -203.0878) (35.3793, -203.1718) (35.3793, -203.236) knots 0 0 0 1 2 2 2
  spline S142 degree 2 poles (35.3793, -203.236) (35.3793, -203.5522) (35.5028, -203.94) (35.5966, -204.0413) knots 0 0 0 1 2 2 2
  spline S143 degree 2 poles (35.5966, -204.0413) (35.6831, -204.1376) (35.8708, -204.2142) (35.977, -204.2142) knots 0 0 0 1 2 2 2
  spline S144 degree 2 poles (35.977, -204.2142) (36.224, -204.2142) (36.5278, -203.8634) (36.5278, -203.5127) knots 0 0 0 1 2 2 2
  point P0 (0, 0)
  constraints: 2 other
emboss "Emboss1" sketch "Sketch13" operation cut depth 2.54 direction (-1, 0, 0)
sketch "Sketch14" plane through (0, 0, 0) normal (-1, 0, 0) x (0, 0, 1)
  line L0 (-10.4499, -187.9273) -> (8.7669, -187.9273) construction
  line L1 (8.7669, -187.9273) -> (8.7669, -196.7101) construction
  line L2 (8.7669, -196.7101) -> (-10.4499, -196.7101) construction
  line L3 (-10.4499, -196.7101) -> (-10.4499, -187.9273) construction
  line L4 (-23.4175, -195.887) -> (-20.8486, -188.267)
  line L5 (-20.8486, -188.267) -> (-19.6013, -188.267)
  line L6 (-19.6013, -188.267) -> (-17.0325, -195.887)
  line L7 (-17.0325, -195.887) -> (-18.1008, -195.887)
  line L8 (-18.1008, -195.887) -> (-18.7924, -193.7566)
  line L9 (-18.7924, -193.7566) -> (-21.7008, -193.7566)
  line L10 (-21.7008, -193.7566) -> (-22.3924, -195.887)
  line L11 (-22.3924, -195.887) -> (-23.4175, -195.887)
  line L12 (-19.0702, -192.8921) -> (-20.2497, -189.3044)
  line L13 (-20.2497, -189.3044) -> (-21.4229, -192.8921)
  line L14 (-21.4229, -192.8921) -> (-19.0702, -192.8921)
  line L15 (-10.4128, -195.887) -> (-11.7281, -195.887)
  line L16 (-11.7281, -195.887) -> (-14.1364, -192.855)
  line L17 (-14.1364, -192.855) -> (-15.2973, -192.855)
  line L18 (-15.2973, -192.855) -> (-15.2973, -195.887)
  line L19 (-15.2973, -195.887) -> (-16.31, -195.887)
  line L20 (-16.31, -195.887) -> (-16.31, -188.267)
  line L21 (-16.31, -188.267) -> (-14.3463, -188.267)
  spline S0 degree 2 poles (-14.3463, -188.267) (-13.6918, -188.267) (-12.8087, -188.409) (-12.4074, -188.6683) knots 0 0 0 1 2 2 2
  spline S1 degree 2 poles (-12.4074, -188.6683) (-12.006, -188.9277) (-11.5429, -189.7366) (-11.5429, -190.3356) knots 0 0 0 1 2 2 2
  spline S2 degree 2 poles (-11.5429, -190.3356) (-11.5429, -191.1692) (-12.395, -192.2993) (-13.1237, -192.571) knots 0 0 0 1 2 2 2
  line L22 (-13.1237, -192.571) -> (-10.4128, -195.887)
  spline S3 degree 2 poles (-12.5988, -190.4159) (-12.5988, -190.0824) (-12.8334, -189.5699) (-13.0804, -189.4032) knots 0 0 0 1 2 2 2
  spline S4 degree 2 poles (-13.0804, -189.4032) (-13.2966, -189.2612) (-13.8708, -189.1438) (-14.2907, -189.1438) knots 0 0 0 1 2 2 2
  line L23 (-14.2907, -189.1438) -> (-15.2973, -189.1438)
  line L24 (-15.2973, -189.1438) -> (-15.2973, -192.009)
  line L25 (-15.2973, -192.009) -> (-14.4081, -192.009)
  spline S5 degree 2 poles (-14.4081, -192.009) (-13.9696, -192.009) (-13.2719, -191.8547) (-13.031, -191.6138) knots 0 0 0 1 2 2 2
  spline S6 degree 2 poles (-13.031, -191.6138) (-12.8087, -191.4039) (-12.5988, -190.8111) (-12.5988, -190.4159) knots 0 0 0 1 2 2 2
  line L26 (-8.0293, -195.887) -> (-8.0293, -189.1685)
  line L27 (-8.0293, -189.1685) -> (-10.5857, -189.1685)
  line L28 (-10.5857, -189.1685) -> (-10.5857, -188.267)
  line L29 (-10.5857, -188.267) -> (-4.4601, -188.267)
  line L30 (-4.4601, -188.267) -> (-4.4601, -189.1685)
  line L31 (-4.4601, -189.1685) -> (-7.0166, -189.1685)
  line L32 (-7.0166, -189.1685) -> (-7.0166, -195.887)
  line L33 (-7.0166, -195.887) -> (-8.0293, -195.887)
  spline S7 degree 2 poles (-1.564, -196.0228) (-2.3914, -196.0228) (-3.5524, -195.677) (-4.0649, -195.43) knots 0 0 0 1 2 2 2
  line L34 (-4.0649, -195.43) -> (-4.0649, -194.158)
  line L35 (-4.0649, -194.158) -> (-3.9908, -194.158)
  spline S8 degree 2 poles (-3.9908, -194.158) (-3.4906, -194.6273) (-2.2247, -195.146) (-1.6381, -195.146) knots 0 0 0 1 2 2 2
  spline S9 degree 2 poles (-1.6381, -195.146) (-0.7983, -195.146) (0.06, -194.4482) (0.06, -193.8739) knots 0 0 0 1 2 2 2
  spline S10 degree 2 poles (0.06, -193.8739) (0.06, -193.417) (-0.3907, -192.8489) (-0.8786, -192.7068) knots 0 0 0 1 2 2 2
  spline S11 degree 2 poles (-0.8786, -192.7068) (-1.2305, -192.608) (-1.8172, -192.4722) (-2.2556, -192.361) knots 0 0 0 1 2 2 2
  spline S12 degree 2 poles (-2.2556, -192.361) (-2.6508, -192.256) (-3.2745, -191.9411) (-3.5153, -191.6879) knots 0 0 0 1 2 2 2
  spline S13 degree 2 poles (-3.5153, -191.6879) (-3.75, -191.4348) (-4.0093, -190.7555) (-4.0093, -190.3109) knots 0 0 0 1 2 2 2
  spline S14 degree 2 poles (-4.0093, -190.3109) (-4.0093, -189.3847) (-2.5643, -188.1311) (-1.4467, -188.1311) knots 0 0 0 1 2 2 2
  spline S15 degree 2 poles (-1.4467, -188.1311) (-0.8045, -188.1311) (0.3317, -188.3843) (0.8196, -188.6251) knots 0 0 0 1 2 2 2
  line L36 (0.8196, -188.6251) -> (0.8196, -189.8354)
  line L37 (0.8196, -189.8354) -> (0.7455, -189.8354)
  spline S16 degree 2 poles (0.7455, -189.8354) (0.3811, -189.502) (-0.7551, -189.008) (-1.3787, -189.008) knots 0 0 0 1 2 2 2
  spline S17 degree 2 poles (-1.3787, -189.008) (-2.0827, -189.008) (-2.9534, -189.6687) (-2.9534, -190.2059) knots 0 0 0 1 2 2 2
  spline S18 degree 2 poles (-2.9534, -190.2059) (-2.9534, -190.6876) (-2.4408, -191.2619) (-1.9592, -191.3915) knots 0 0 0 1 2 2 2
  spline S19 degree 2 poles (-1.9592, -191.3915) (-1.6381, -191.478) (-0.7057, -191.7003) (-0.3969, -191.7929) knots 0 0 0 1 2 2 2
  spline S20 degree 2 poles (-0.3969, -191.7929) (0.3873, -192.0337) (1.116, -193.0032) (1.116, -193.7134) knots 0 0 0 1 2 2 2
  spline S21 degree 2 poles (1.116, -193.7134) (1.116, -194.1641) (0.7516, -195.0286) (0.4244, -195.3312) knots 0 0 0 1 2 2 2
  spline S22 degree 2 poles (0.4244, -195.3312) (0.06, -195.6647) (-0.8662, -196.0228) (-1.564, -196.0228) knots 0 0 0 1 2 2 2
  line L38 (4.7222, -193.0156) -> (1.8385, -193.0156)
  line L39 (1.8385, -193.0156) -> (1.8385, -192.0893)
  line L40 (1.8385, -192.0893) -> (4.7222, -192.0893)
  line L41 (4.7222, -192.0893) -> (4.7222, -193.0156)
  line L42 (10.3662, -195.887) -> (5.951, -195.887)
  line L43 (5.951, -195.887) -> (5.951, -188.267)
  line L44 (5.951, -188.267) -> (6.9637, -188.267)
  line L45 (6.9637, -188.267) -> (6.9637, -194.9854)
  line L46 (6.9637, -194.9854) -> (10.3662, -194.9854)
  line L47 (10.3662, -194.9854) -> (10.3662, -195.887)
  spline S23 degree 2 poles (14.275, -195.2818) (14.1577, -195.3683) (13.7625, -195.677) (13.5772, -195.7696) knots 0 0 0 1 2 2 2
  spline S24 degree 2 poles (13.5772, -195.7696) (13.324, -195.9055) (12.8486, -196.0475) (12.4163, -196.0475) knots 0 0 0 1 2 2 2
  spline S25 degree 2 poles (12.4163, -196.0475) (12.0643, -196.0475) (11.4283, -195.782) (11.1875, -195.5412) knots 0 0 0 1 2 2 2
  spline S26 degree 2 poles (11.1875, -195.5412) (10.959, -195.3065) (10.6811, -194.6149) (10.6811, -194.2321) knots 0 0 0 1 2 2 2
  spline S27 degree 2 poles (10.6811, -194.2321) (10.6811, -193.6393) (11.1813, -192.7995) (11.7247, -192.5586) knots 0 0 0 1 2 2 2
  spline S28 degree 2 poles (11.7247, -192.5586) (12.2063, -192.3363) (13.5155, -192.1696) (14.275, -192.1264) knots 0 0 0 1 2 2 2
  line L48 (14.275, -192.1264) -> (14.275, -191.9411)
  spline S29 degree 2 poles (14.275, -191.9411) (14.275, -191.6077) (14.0712, -191.1939) (13.886, -191.0766) knots 0 0 0 1 2 2 2
  spline S30 degree 2 poles (13.886, -191.0766) (13.7007, -190.9593) (13.1697, -190.8852) (12.8856, -190.8852) knots 0 0 0 1 2 2 2
  spline S31 degree 2 poles (12.8856, -190.8852) (12.5522, -190.8852) (11.6506, -191.0828) (11.1998, -191.2742) knots 0 0 0 1 2 2 2
  line L49 (11.1998, -191.2742) -> (11.1442, -191.2742)
  line L50 (11.1442, -191.2742) -> (11.1442, -190.2924)
  spline S32 degree 2 poles (11.1442, -190.2924) (11.4098, -190.2183) (12.404, -190.033) (12.8918, -190.033) knots 0 0 0 1 2 2 2
  spline S33 degree 2 poles (12.8918, -190.033) (13.4846, -190.033) (14.2935, -190.2183) (14.6146, -190.4591) knots 0 0 0 1 2 2 2
  spline S34 degree 2 poles (14.6146, -190.4591) (14.9295, -190.6938) (15.2383, -191.4409) (15.2383, -191.9782) knots 0 0 0 1 2 2 2
  line L51 (15.2383, -191.9782) -> (15.2383, -195.887)
  line L52 (15.2383, -195.887) -> (14.275, -195.887)
  line L53 (14.275, -195.887) -> (14.275, -195.2818)
  line L54 (14.275, -194.4791) -> (14.275, -192.8921)
  spline S35 degree 2 poles (14.275, -192.8921) (13.9292, -192.923) (12.8856, -193.0279) (12.5583, -193.1267) knots 0 0 0 1 2 2 2
  spline S36 degree 2 poles (12.5583, -193.1267) (12.1755, -193.2441) (11.6753, -193.7319) (11.6753, -194.1641) knots 0 0 0 1 2 2 2
  spline S37 degree 2 poles (11.6753, -194.1641) (11.6753, -194.6581) (12.231, -195.1583) (12.7621, -195.1583) knots 0 0 0 1 2 2 2
  spline S38 degree 2 poles (12.7621, -195.1583) (13.2129, -195.1583) (13.9539, -194.7693) (14.275, -194.4791) knots 0 0 0 1 2 2 2
  spline S39 degree 2 poles (21.3825, -192.9353) (21.3825, -194.337) (20.024, -196.0475) (18.9989, -196.0475) knots 0 0 0 1 2 2 2
  spline S40 degree 2 poles (18.9989, -196.0475) (18.5358, -196.0475) (17.875, -195.819) (17.5539, -195.6214) knots 0 0 0 1 2 2 2
  line L55 (17.5539, -195.6214) -> (17.4922, -195.887)
  line L56 (17.4922, -195.887) -> (16.5906, -195.887)
  line L57 (16.5906, -195.887) -> (16.5906, -187.9273)
  line L58 (16.5906, -187.9273) -> (17.5539, -187.9273)
  line L59 (17.5539, -187.9273) -> (17.5539, -190.7679)
  spline S41 degree 2 poles (17.5539, -190.7679) (17.9183, -190.4406) (18.7642, -190.0083) (19.3015, -190.0083) knots 0 0 0 1 2 2 2
  spline S42 degree 2 poles (19.3015, -190.0083) (20.271, -190.0083) (21.3825, -191.5583) (21.3825, -192.9353) knots 0 0 0 1 2 2 2
  spline S43 degree 2 poles (20.3883, -193.0094) (20.3883, -191.9843) (19.7646, -190.9222) (19.073, -190.9222) knots 0 0 0 1 2 2 2
  spline S44 degree 2 poles (19.073, -190.9222) (18.684, -190.9222) (17.8812, -191.2927) (17.5539, -191.5768) knots 0 0 0 1 2 2 2
  line L60 (17.5539, -191.5768) -> (17.5539, -194.8557)
  spline S45 degree 2 poles (17.5539, -194.8557) (17.9183, -195.0348) (18.4802, -195.183) (18.8136, -195.183) knots 0 0 0 1 2 2 2
  spline S46 degree 2 poles (18.8136, -195.183) (19.5485, -195.183) (20.3883, -194.1394) (20.3883, -193.0094) knots 0 0 0 1 2 2 2
  point P0 (0, 0)
  constraints: 2 other
emboss "Emboss2" sketch "Sketch14" operation cut depth 2.54 direction (1, 0, 0)
sketch "Sketch15" plane through (0, -213.7841, 48.4212) normal (0, 0, 1) x (1, 0, 0)
  line L0 (20.32, 0) -> (20.32, 261.366) projected
  line L1 (16.002, 162.687) -> (20.32, 162.687)
  line L2 (20.32, 162.687) -> (20.32, 170.688)
  line L3 (20.32, 170.688) -> (16.002, 170.688)
  line L4 (16.002, 170.688) -> (16.002, 162.687)
  line L5 (20.32, 264.541) -> (0, 264.541) projected
  point P0 (0, 213.7841)
  point P1 (18.161, 170.688)
  dimension "d78" = 8.001
  dimension "d79" = 4.318
  dimension "d83" = 101.854
  constraints: 8 end point, 2 parallel, 1 horizontal, 1 midpoint, 1 perpendicular, 1 point on line
  measures "d78" distance of L3.end L1.start
  measures "d79" distance between parallel lines of L0 L4
  measures "d83" distance between parallel lines of L5 L1
extrude "Extrusion9" cut sketch "Sketch15" against normal blind 6.35
sketch "Sketch18" plane through (0, -216.9591, -50.0038) normal (0, -1, 0) x (1, 0, 0)
  line L0 (20.32, 43.2816) -> (20.32, 53.2892)
  line L1 (20.32, 53.2892) -> (19.1008, 53.2892)
  line L2 (19.1008, 53.2892) -> (17.3482, 51.2892)
  line L3 (17.3482, 45.2816) -> (17.3482, 51.2892)
  line L4 (20.32, 98.425) -> (0, 98.425) projected
  line L5 (20.32, 95.25) -> (20.32, 0) projected
  line L6 (20.32, 43.2816) -> (19.1008, 43.2816)
  line L7 (19.1008, 43.2816) -> (17.3482, 45.2816)
  point P0 (19.7104, 53.2892)
  dimension "d91" = 1.2192
  dimension "d92" = 2
  dimension "d94" = 6.0076
  dimension "d95" = 10.0076
  dimension "d98" = 1.7526
  dimension "d99" = 0
  dimension "d165" = 45.1358
  constraints: 12 end point, 1 horizontal, 1 midpoint
  measures "d91" distance of L0.end L1.end
  measures "d92" vertical distance of L1.end L2.end
  measures "d94" distance of L3.start L2.end
  measures "d95" distance of L0.start L0.end
  measures "d98" distance from line of L1.end L3
  measures "d99" distance between parallel lines of L5 L0
  measures "d165" distance from line of L4 point (19.71, 53.289)
extrude "Extrusion10" cut sketch "Sketch18" against normal blind 6.35
sketch "Sketch19" plane through (0, 13.9785, -4.7779) normal (-1, 0, 0) x (0, 0, 1)
  arc A0 (-41.5361, 32.5875) -> (-44.2099, 29.9137) centre (-43.3209, 31.6985) ccw projected
  circle A1 centre (-43.3209, 31.6985) radius 4.5085
  arc A2 (46.3344, 32.5875) -> (49.0081, 29.9137) centre (48.1191, 31.6985) ccw projected
  circle A3 centre (48.1191, 31.6985) radius 4.5085
  circle A4 centre (-43.3209, -225.8575) radius 1.9939 projected
  circle A5 centre (-43.3209, -225.8575) radius 4.5085
  arc A6 (46.3164, -226.7095) -> (48.9711, -224.0548) centre (48.1191, -225.8575) ccw projected
  circle A7 centre (48.1191, -225.8575) radius 4.5085
  circle A8 centre (-38.2409, -77.5215) radius 4.5085
  circle A9 centre (-38.2409, -77.5215) radius 1.9939 projected
  circle A10 centre (43.0391, -77.5215) radius 4.5085
  circle A11 centre (43.0391, -77.5215) radius 1.9939 projected
  point P0 (0, 0)
  dimension "d110" = 9.017
  dimension "d111" = 9.017
  dimension "d112" = 9.017
  dimension "d113" = 9.017
  dimension "d120" = 9.017
  dimension "d121" = 0
  dimension "d122" = 0
  dimension "d123" = 9.017
  dimension "d124" = 0
  dimension "d125" = 0
  constraints: 6 centre point, 4 coincident
  measures "d110" diameter of A1
  measures "d111" diameter of A3
  measures "d112" diameter of A5
  measures "d113" diameter of A7
  measures "d120" diameter of A8
  measures "d121" distance of A9.centre A8.centre
  measures "d122" distance of A9.centre A8.centre
  measures "d123" diameter of A10
  measures "d124" distance of A11.centre A10.centre
  measures "d125" distance of A11.centre A10.centre
extrude "Extrusion11" cut sketch "Sketch19" against normal blind 5 contours A1 | A3 | A4 | A5 | A7 | A8 | A9 | A10 | A11
sketch "Sketch20" plane through (0, -216.9591, -50.0038) normal (0, -1, 0) x (1, 0, 0)
  circle A0 centre (18.288, 65.4174) radius 2.032
  line L0 (20.32, 98.425) -> (0, 98.425) projected
  line L1 (20.32, 95.25) -> (20.32, 53.2892) projected
  point P0 (0, 50.0038)
  dimension "d126" = 4.064
  dimension "d127" = 33.0076
  dimension "d128" = 2.032
  constraints: 1 centre point
  measures "d126" diameter of A0
  measures "d127" distance from line of L0 A0.centre
  measures "d128" distance from line of L1 A0.centre
extrude "Extrusion12" cut sketch "Sketch20" against normal blind 13.97